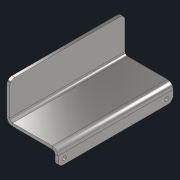
# Autodesk Inventor part: plate7
Saved by Autodesk Inventor 2021 (Build 250183000, 183)
## iProperties
Created: 2021-07-24
Part Number: plate7
Material: 鋼、炭素鋼
Document SubType Name: Sheet Metal
Designer: yuta0
Density: 7.85 g/cm^3
Sheet Metal Rule: Default_mm
Appearance: 半つや出し
購入先: Meviy
在庫数: 0.0
Author: yuta0
Autodesk Inventor part; units mm, degrees
ref_plane "YZ Plane" through (0, 0, 0) normal (1, 0, 0) x (0, 1, 0)
ref_plane "XZ Plane" through (0, 0, 0) normal (0, 1, 0) x (-1, 0, 0)
ref_plane "XY Plane" through (0, 0, 0) normal (0, 0, 1) x (1, 0, 0)
sketch "スケッチ1" plane through (0, 0, 0) normal (0, 1, 0) x (-1, 0, 0)
  line L0 (-20, 45) -> (20, 45)
  line L1 (20, 45) -> (20, -45)
  line L2 (20, -45) -> (-20, -45)
  line L3 (-20, -45) -> (-20, 45)
  line L4 (-20, 45) -> (20, -45) construction
  line L5 (20, 45) -> (-20, -45) construction
  point P0 (0, 0)
  dimension "d0" = 90
  dimension "d1" = 40
  measures "d0" distance of L0.end L1.end
  measures "d1" distance of L0.start L0.end
extrude "プレート1" add sketch "スケッチ1" along normal blind 2.3
sketch "スケッチ2" plane through (17.7, 2.3, 45) normal (1, 0, 0) x (0, 1, 0)
  line L0 (0, -90) -> (0, 0)
  line L1 (0, 0) -> (-12.6, 0)
  line L2 (-12.6, 0) -> (-12.6, -90)
  line L3 (-12.6, -90) -> (0, -90)
  constraints: 6 end point, 1 horizontal, 1 perpendicular, 1 vertical
edge flange "フランジ1" height 12.6 angle 90 thickness 2.3 bend radius 2.3 thickness toward (1, 0, 0) relief straight relief width 2.3 relief depth 1.15 edges at (20, 0, 0) wall of the first edge with corners at (17.7, 2.3, -45) (17.7, 2.3, 45) (17.7, -10.3, 45) (17.7, -10.3, -45)
bend "曲げ1"
corner "コーナー1"
sketch "スケッチ3" plane through (-17.7, 0, 45) normal (-1, 0, 0) x (0, -1, 0)
  line L0 (0, -90) -> (0, 0)
  line L1 (0, 0) -> (-30, 0)
  line L2 (-30, 0) -> (-30, -90)
  line L3 (-30, -90) -> (0, -90)
  constraints: 6 end point, 1 horizontal, 1 perpendicular, 1 vertical
edge flange "フランジ2" height 30 angle 90 thickness 2.3 bend radius 2.3 thickness toward (-1, 0, 0) relief straight relief width 2.3 relief depth 1.15 edges at (-20, 2.3, 0) wall of the first edge with corners at (-17.7, 0, -45) (-17.7, 0, 45) (-17.7, 30, 45) (-17.7, 30, -45)
bend "曲げ2"
corner "コーナー2"
sketch "スケッチ4" plane through (20, -10.3, 45) normal (1, 0, 0) x (0, 0, -1)
  line L0 (90, 0) -> (0, 0) projected
  line L1 (0, 0) -> (0, 8) projected
  point P0 (45, 10.3)
  point P1 (5, 4)
  point P2 (85, 4)
  dimension "d23" = 4
  dimension "d24" = 80
  dimension "d25" = 5
  constraints: 1 horizontal alignment
  measures "d23" distance from line of L0 point (5, 4)
  measures "d24" distance of point (85, 4) point (5, 4)
  measures "d25" distance from line of L1 point (5, 4)
hole "穴1" at (20, -6.3, 40) at (20, -6.3, -40) direction (-1, 0, 0) diameter 3.2 depth 2.3 tip angle 118 clearance for "Flat Head Machine Screw" size "M3" standard "Ansi Metric M Profile"
fillet "コーナーR1" radius 4 4 edges at (18.85, -10.3, 45) (18.85, -10.3, -45) (-18.85, 30, 45) (-18.85, 30, -45)
equation "\"d31\" = Thickness"
equation "\"d2\" = Thickness"
equation "\"d3\" = BendReliefWidth"
equation "\"d4\" = BendReliefDepth"
equation "\"d5\" = MinimumRemnant"
equation "\"d6\" = TransitionRadius"
equation "\"d9\" = BendRadius"
equation "\"d10\" = CornerReliefSize"
equation "\"d11\" = GapSize"
equation "\"d12\" = JacobiRadiusSize"
equation "\"d13\" = BendReliefWidth"
equation "\"d14\" = BendReliefDepth"
equation "\"d15\" = MinimumRemnant"
equation "\"d16\" = TransitionRadius"
equation "\"d19\" = BendRadius"
equation "\"d20\" = CornerReliefSize"
equation "\"d21\" = GapSize"
equation "\"d22\" = JacobiRadiusSize"
equation "\"BendRadius\" = Thickness"
equation "\"BendReliefWidth\" = Thickness"
equation "\"BendReliefDepth\" = 0.5 * Thickness"
equation "\"CornerReliefSize\" = 4 * Thickness"
equation "\"MinimumRemnant\" = 2 * Thickness"
equation "\"TransitionRadius\" = BendRadius"
equation "\"JacobiRadiusSize\" = BendRadius"
equation "\"GapSize\" = Thickness"
equation "\"Thickness\" = 2.3"
